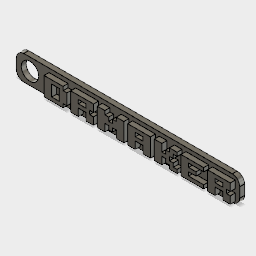
drmaker_big v0 (Autodesk Fusion 360 design; units mm, degrees)
Autodesk Fusion 360 part; units mm, degrees
sketch "Base" plane through (0, 0, 0) normal (0, 0, 1) x (1, 0, 0)
  line L0 (-45, 5) -> (45, 5)
  line L1 (45, 5) -> (45, -5)
  line L2 (45, -5) -> (-45, -5)
  line L3 (-45, -5) -> (-45, 5)
  line L4 (-45, 5) -> (45, -5) construction
  line L5 (45, 5) -> (-45, -5) construction
  dimension "d1" = 10
  dimension "d2" = 90
  constraint perpendicular L0 L1
  constraint parallel L0 L2
  constraint parallel L1 L3
  constraint horizontal L0
  constraint coincident L4 origin
  constraint coincident L5 origin
extrude "Extrude1" add sketch "Base" along normal blind 2
sketch "Text" plane through (0, 0, 2) normal (0, 0, 1) x (1, 0, 0)
  line L0 (-45, -5) -> (45, -5)
  line L1 (45, -5) -> (45, 5)
  line L2 (45, 5) -> (-45, 5)
  line L3 (-45, 5) -> (-45, -5)
  line L4 (-31.801, -4.0707) -> (-24.1511, -4.0707)
  line L5 (-24.1511, -4.0707) -> (-24.1511, -2.5707)
  line L6 (-24.1511, -2.5707) -> (-22.6212, -2.5707)
  line L7 (-22.6212, -2.5707) -> (-22.6212, 1.9293)
  line L8 (-22.6212, 1.9293) -> (-24.1511, 1.9293)
  line L9 (-24.1511, 1.9293) -> (-24.1511, 3.4293)
  line L10 (-24.1511, 3.4293) -> (-31.801, 3.4293)
  line L11 (-31.801, 3.4293) -> (-31.801, -4.0707)
  line L12 (-28.741, 1.9293) -> (-25.6811, 1.9293)
  line L13 (-25.6811, 1.9293) -> (-25.6811, -2.5707)
  line L14 (-25.6811, -2.5707) -> (-28.741, -2.5707)
  line L15 (-28.741, -2.5707) -> (-28.741, 1.9293)
  line L16 (-18.0233, -1.0707) -> (-14.9634, -1.0707)
  line L17 (-14.9634, -1.0707) -> (-14.9634, -4.0707)
  line L18 (-14.9634, -4.0707) -> (-11.9035, -4.0707)
  line L19 (-11.9035, -4.0707) -> (-11.9035, -1.0707)
  line L20 (-11.9035, -1.0707) -> (-13.4334, -1.0707)
  line L21 (-13.4334, -1.0707) -> (-13.4334, 0.4293)
  line L22 (-13.4334, 0.4293) -> (-11.9035, 0.4293)
  line L23 (-11.9035, 0.4293) -> (-11.9035, 3.4293)
  line L24 (-11.9035, 3.4293) -> (-21.0833, 3.4293)
  line L25 (-21.0833, 3.4293) -> (-21.0833, -4.0707)
  line L26 (-21.0833, -4.0707) -> (-18.0233, -4.0707)
  line L27 (-18.0233, -4.0707) -> (-18.0233, -1.0707)
  line L28 (-18.0233, 1.9293) -> (-14.9634, 1.9293)
  line L29 (-14.9634, 1.9293) -> (-14.9634, 0.4293)
  line L30 (-14.9634, 0.4293) -> (-18.0233, 0.4293)
  line L31 (-18.0233, 0.4293) -> (-18.0233, 1.9293)
  line L32 (-7.3056, -1.0707) -> (-5.7757, -1.0707)
  line L33 (-5.7757, -1.0707) -> (-5.7757, -2.5707)
  line L34 (-5.7757, -2.5707) -> (-4.2457, -2.5707)
  line L35 (-4.2457, -2.5707) -> (-4.2457, -1.0707)
  line L36 (-4.2457, -1.0707) -> (-2.7157, -1.0707)
  line L37 (-2.7157, -1.0707) -> (-2.7157, -4.0707)
  line L38 (-2.7157, -4.0707) -> (0.3442, -4.0707)
  line L39 (0.3442, -4.0707) -> (0.3442, 3.4293)
  line L40 (0.3442, 3.4293) -> (-2.7157, 3.4293)
  line L41 (-2.7157, 3.4293) -> (-2.7157, 1.9293)
  line L42 (-2.7157, 1.9293) -> (-4.2457, 1.9293)
  line L43 (-4.2457, 1.9293) -> (-4.2457, 0.4293)
  line L44 (-4.2457, 0.4293) -> (-5.7757, 0.4293)
  line L45 (-5.7757, 0.4293) -> (-5.7757, 1.9293)
  line L46 (-5.7757, 1.9293) -> (-7.3056, 1.9293)
  line L47 (-7.3056, 1.9293) -> (-7.3056, 3.4293)
  line L48 (-7.3056, 3.4293) -> (-10.3656, 3.4293)
  line L49 (-10.3656, 3.4293) -> (-10.3656, -4.0707)
  line L50 (-10.3656, -4.0707) -> (-7.3056, -4.0707)
  line L51 (-7.3056, -4.0707) -> (-7.3056, -1.0707)
  line L52 (4.9261, -1.0707) -> (7.986, -1.0707)
  line L53 (7.986, -1.0707) -> (7.986, -4.0707)
  line L54 (7.986, -4.0707) -> (11.0459, -4.0707)
  line L55 (11.0459, -4.0707) -> (11.0459, 3.4293)
  line L56 (11.0459, 3.4293) -> (1.8662, 3.4293)
  line L57 (1.8662, 3.4293) -> (1.8662, -4.0707)
  line L58 (1.8662, -4.0707) -> (4.9261, -4.0707)
  line L59 (4.9261, -4.0707) -> (4.9261, -1.0707)
  line L60 (4.9261, 1.9293) -> (7.986, 1.9293)
  line L61 (7.986, 1.9293) -> (7.986, 0.4293)
  line L62 (7.986, 0.4293) -> (4.9261, 0.4293)
  line L63 (4.9261, 0.4293) -> (4.9261, 1.9293)
  line L64 (15.6438, -1.0707) -> (17.1738, -1.0707)
  line L65 (17.1738, -1.0707) -> (17.1738, -2.5707)
  line L66 (17.1738, -2.5707) -> (18.7037, -2.5707)
  line L67 (18.7037, -2.5707) -> (18.7037, -4.0707)
  line L68 (18.7037, -4.0707) -> (21.7636, -4.0707)
  line L69 (21.7636, -4.0707) -> (21.7636, -2.5707)
  line L70 (21.7636, -2.5707) -> (20.2337, -2.5707)
  line L71 (20.2337, -2.5707) -> (20.2337, -1.0707)
  line L72 (20.2337, -1.0707) -> (18.7037, -1.0707)
  line L73 (18.7037, -1.0707) -> (18.7037, 0.4293)
  line L74 (18.7037, 0.4293) -> (20.2337, 0.4293)
  line L75 (20.2337, 0.4293) -> (20.2337, 1.9293)
  line L76 (20.2337, 1.9293) -> (21.7636, 1.9293)
  line L77 (21.7636, 1.9293) -> (21.7636, 3.4293)
  line L78 (21.7636, 3.4293) -> (18.7037, 3.4293)
  line L79 (18.7037, 3.4293) -> (18.7037, 1.9293)
  line L80 (18.7037, 1.9293) -> (17.1738, 1.9293)
  line L81 (17.1738, 1.9293) -> (17.1738, 0.4293)
  line L82 (17.1738, 0.4293) -> (15.6438, 0.4293)
  line L83 (15.6438, 0.4293) -> (15.6438, 3.4293)
  line L84 (15.6438, 3.4293) -> (12.5839, 3.4293)
  line L85 (12.5839, 3.4293) -> (12.5839, -4.0707)
  line L86 (12.5839, -4.0707) -> (15.6438, -4.0707)
  line L87 (15.6438, -4.0707) -> (15.6438, -1.0707)
  line L88 (23.3016, -4.0707) -> (32.4813, -4.0707)
  line L89 (32.4813, -4.0707) -> (32.4813, -2.5707)
  line L90 (32.4813, -2.5707) -> (26.3615, -2.5707)
  line L91 (26.3615, -2.5707) -> (26.3615, -1.0707)
  line L92 (26.3615, -1.0707) -> (29.4214, -1.0707)
  line L93 (29.4214, -1.0707) -> (29.4214, 0.4293)
  line L94 (29.4214, 0.4293) -> (26.3615, 0.4293)
  line L95 (26.3615, 0.4293) -> (26.3615, 1.9293)
  line L96 (26.3615, 1.9293) -> (32.4813, 1.9293)
  line L97 (32.4813, 1.9293) -> (32.4813, 3.4293)
  line L98 (32.4813, 3.4293) -> (23.3016, 3.4293)
  line L99 (23.3016, 3.4293) -> (23.3016, -4.0707)
  line L100 (37.0792, -1.0707) -> (40.1391, -1.0707)
  line L101 (40.1391, -1.0707) -> (40.1391, -4.0707)
  line L102 (40.1391, -4.0707) -> (43.199, -4.0707)
  line L103 (43.199, -4.0707) -> (43.199, -1.0707)
  line L104 (43.199, -1.0707) -> (41.6691, -1.0707)
  line L105 (41.6691, -1.0707) -> (41.6691, 0.4293)
  line L106 (41.6691, 0.4293) -> (43.199, 0.4293)
  line L107 (43.199, 0.4293) -> (43.199, 3.4293)
  line L108 (43.199, 3.4293) -> (34.0193, 3.4293)
  line L109 (34.0193, 3.4293) -> (34.0193, -4.0707)
  line L110 (34.0193, -4.0707) -> (37.0792, -4.0707)
  line L111 (37.0792, -4.0707) -> (37.0792, -1.0707)
  line L112 (37.0792, 1.9293) -> (40.1391, 1.9293)
  line L113 (40.1391, 1.9293) -> (40.1391, 0.4293)
  line L114 (40.1391, 0.4293) -> (37.0792, 0.4293)
  line L115 (37.0792, 0.4293) -> (37.0792, 1.9293)
extrude "Extrude2" add sketch "Text" along normal blind 2 contours L4 L5 L6 L7 L8 L9 L10 L11 | L16 L17 L18 L19 L20 L21 L22 L23 L24 L25 L26 L27 | L32 L33 L34 L35 L36 L37 L38 L39 L40 L41 L42 L43 L44 L45 L46 L47 L48 L49 L50 L51 | L52 L53 L54 L55 L56 L57 L58 L59 | L64 L65 L66 L67 L68 L69 L70 L71 L72 L73 L74 L75 L76 L77 L78 L79 L80 L81 L82 L83 L84 L85 L86 L87 | L88 L89 L90 L91 L92 L93 L94 L95 L96 L97 L98 L99 | L100 L101 L102 L103 L104 L105 L106 L107 L108 L109 L110 L111
fillet "Fillet1" radius 3 4 edges at (45, 5, 1) (45, -5, 1) (-45, -5, 1) (-45, 5, 1)
sketch "Sketch3" plane through (0, 0, 2) normal (0, 0, 1) x (1, 0, 0)
  line L0 (-18.0233, -4.0707) -> (-21.0833, -4.0707)
  line L1 (-21.0833, -4.0707) -> (-21.0833, 3.4293)
  line L2 (-21.0833, 3.4293) -> (-11.9035, 3.4293)
  line L3 (-11.9035, 3.4293) -> (-11.9035, 0.4293)
  line L4 (-11.9035, 0.4293) -> (-13.4334, 0.4293)
  line L5 (-13.4334, 0.4293) -> (-13.4334, -1.0707)
  line L6 (-13.4334, -1.0707) -> (-11.9035, -1.0707)
  line L7 (-11.9035, -1.0707) -> (-11.9035, -4.0707)
  line L8 (-11.9035, -4.0707) -> (-14.9634, -4.0707)
  line L9 (-14.9634, -4.0707) -> (-14.9634, -1.0707)
  line L10 (-14.9634, -1.0707) -> (-18.0233, -1.0707)
  line L11 (-18.0233, -1.0707) -> (-18.0233, -4.0707)
  line L12 (23.3016, 3.4293) -> (32.4813, 3.4293)
  line L13 (32.4813, 3.4293) -> (32.4813, 1.9293)
  line L14 (32.4813, 1.9293) -> (26.3615, 1.9293)
  line L15 (26.3615, 1.9293) -> (26.3615, 0.4293)
  line L16 (26.3615, 0.4293) -> (29.4214, 0.4293)
  line L17 (29.4214, 0.4293) -> (29.4214, -1.0707)
  line L18 (29.4214, -1.0707) -> (26.3615, -1.0707)
  line L19 (26.3615, -1.0707) -> (26.3615, -2.5707)
  line L20 (26.3615, -2.5707) -> (32.4813, -2.5707)
  line L21 (32.4813, -2.5707) -> (32.4813, -4.0707)
  line L22 (32.4813, -4.0707) -> (23.3016, -4.0707)
  line L23 (23.3016, -4.0707) -> (23.3016, 3.4293)
  line L24 (-31.801, 3.4293) -> (-24.1511, 3.4293)
  line L25 (-24.1511, 3.4293) -> (-24.1511, 1.9293)
  line L26 (-24.1511, 1.9293) -> (-22.6212, 1.9293)
  line L27 (-22.6212, 1.9293) -> (-22.6212, -2.5707)
  line L28 (-22.6212, -2.5707) -> (-24.1511, -2.5707)
  line L29 (-24.1511, -2.5707) -> (-24.1511, -4.0707)
  line L30 (-24.1511, -4.0707) -> (-31.801, -4.0707)
  line L31 (-31.801, -4.0707) -> (-31.801, 3.4293)
  line L32 (15.6438, -4.0707) -> (12.5839, -4.0707)
  line L33 (12.5839, -4.0707) -> (12.5839, 3.4293)
  line L34 (12.5839, 3.4293) -> (15.6438, 3.4293)
  line L35 (15.6438, 3.4293) -> (15.6438, 0.4293)
  line L36 (15.6438, 0.4293) -> (17.1738, 0.4293)
  line L37 (17.1738, 0.4293) -> (17.1738, 1.9293)
  line L38 (17.1738, 1.9293) -> (18.7037, 1.9293)
  line L39 (18.7037, 1.9293) -> (18.7037, 3.4293)
  line L40 (18.7037, 3.4293) -> (21.7636, 3.4293)
  line L41 (21.7636, 3.4293) -> (21.7636, 1.9293)
  line L42 (21.7636, 1.9293) -> (20.2337, 1.9293)
  line L43 (20.2337, 1.9293) -> (20.2337, 0.4293)
  line L44 (20.2337, 0.4293) -> (18.7037, 0.4293)
  line L45 (18.7037, 0.4293) -> (18.7037, -1.0707)
  line L46 (18.7037, -1.0707) -> (20.2337, -1.0707)
  line L47 (20.2337, -1.0707) -> (20.2337, -2.5707)
  line L48 (20.2337, -2.5707) -> (21.7636, -2.5707)
  line L49 (21.7636, -2.5707) -> (21.7636, -4.0707)
  line L50 (21.7636, -4.0707) -> (18.7037, -4.0707)
  line L51 (18.7037, -4.0707) -> (18.7037, -2.5707)
  line L52 (18.7037, -2.5707) -> (17.1738, -2.5707)
  line L53 (17.1738, -2.5707) -> (17.1738, -1.0707)
  line L54 (17.1738, -1.0707) -> (15.6438, -1.0707)
  line L55 (15.6438, -1.0707) -> (15.6438, -4.0707)
  arc A0 (-42, 5) -> (-45, 2) centre (-42, 2) ccw
  line L56 (-45, 2) -> (-45, -2)
  arc A1 (-45, -2) -> (-42, -5) centre (-42, -2) ccw
  line L57 (-42, -5) -> (42, -5)
  arc A2 (42, -5) -> (45, -2) centre (42, -2) ccw
  line L58 (45, -2) -> (45, 2)
  arc A3 (45, 2) -> (42, 5) centre (42, 2) ccw
  line L59 (42, 5) -> (-42, 5)
  line L60 (4.9261, -4.0707) -> (1.8662, -4.0707)
  line L61 (1.8662, -4.0707) -> (1.8662, 3.4293)
  line L62 (1.8662, 3.4293) -> (11.0459, 3.4293)
  line L63 (11.0459, 3.4293) -> (11.0459, -4.0707)
  line L64 (11.0459, -4.0707) -> (7.986, -4.0707)
  line L65 (7.986, -4.0707) -> (7.986, -1.0707)
  line L66 (7.986, -1.0707) -> (4.9261, -1.0707)
  line L67 (4.9261, -1.0707) -> (4.9261, -4.0707)
  line L68 (-7.3056, -4.0707) -> (-10.3656, -4.0707)
  line L69 (-10.3656, -4.0707) -> (-10.3656, 3.4293)
  line L70 (-10.3656, 3.4293) -> (-7.3056, 3.4293)
  line L71 (-7.3056, 3.4293) -> (-7.3056, 1.9293)
  line L72 (-7.3056, 1.9293) -> (-5.7757, 1.9293)
  line L73 (-5.7757, 1.9293) -> (-5.7757, 0.4293)
  line L74 (-5.7757, 0.4293) -> (-4.2457, 0.4293)
  line L75 (-4.2457, 0.4293) -> (-4.2457, 1.9293)
  line L76 (-4.2457, 1.9293) -> (-2.7157, 1.9293)
  line L77 (-2.7157, 1.9293) -> (-2.7157, 3.4293)
  line L78 (-2.7157, 3.4293) -> (0.3442, 3.4293)
  line L79 (0.3442, 3.4293) -> (0.3442, -4.0707)
  line L80 (0.3442, -4.0707) -> (-2.7157, -4.0707)
  line L81 (-2.7157, -4.0707) -> (-2.7157, -1.0707)
  line L82 (-2.7157, -1.0707) -> (-4.2457, -1.0707)
  line L83 (-4.2457, -1.0707) -> (-4.2457, -2.5707)
  line L84 (-4.2457, -2.5707) -> (-5.7757, -2.5707)
  line L85 (-5.7757, -2.5707) -> (-5.7757, -1.0707)
  line L86 (-5.7757, -1.0707) -> (-7.3056, -1.0707)
  line L87 (-7.3056, -1.0707) -> (-7.3056, -4.0707)
  line L88 (37.0792, -4.0707) -> (34.0193, -4.0707)
  line L89 (34.0193, -4.0707) -> (34.0193, 3.4293)
  line L90 (34.0193, 3.4293) -> (43.199, 3.4293)
  line L91 (43.199, 3.4293) -> (43.199, 0.4293)
  line L92 (43.199, 0.4293) -> (41.6691, 0.4293)
  line L93 (41.6691, 0.4293) -> (41.6691, -1.0707)
  line L94 (41.6691, -1.0707) -> (43.199, -1.0707)
  line L95 (43.199, -1.0707) -> (43.199, -4.0707)
  line L96 (43.199, -4.0707) -> (40.1391, -4.0707)
  line L97 (40.1391, -4.0707) -> (40.1391, -1.0707)
  line L98 (40.1391, -1.0707) -> (37.0792, -1.0707)
  line L99 (37.0792, -1.0707) -> (37.0792, -4.0707)
  circle A4 centre (-39.5, 0) radius 3.5
  dimension "d8" = 7
  dimension "d9" = 5.5
  measures "d8" diameter of A4
extrude "Extrude3" cut sketch "Sketch3" against normal through all contours A4
